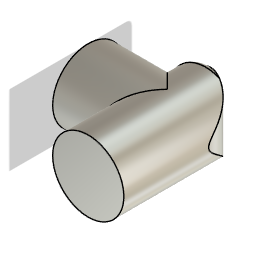
Link5 v14 (Autodesk Fusion 360 design; units mm, degrees)
Autodesk Fusion 360 part; units mm, degrees
sketch "Boceto1" plane through (0, 0, 0) normal (0, 0, 1) x (1, 0, 0)
  circle A0 centre (0, 0) radius 45
  circle A1 centre (0, 0) radius 30
  dimension "d1" = 90
  dimension "d12" = 60
  constraint coincident A0.centre A1.centre
  measures "d1" diameter of A0
  measures "d12" diameter of A1
extrude "Extruir1" add sketch "Boceto1" along normal blind 100 contours A0 | A1
sketch "Boceto2" plane through (0, 0, 0) normal (1, 0, 0) x (0, 0, -1)
  circle A0 centre (0, 0) radius 45
  circle A1 centre (0, 0) radius 32.5
  dimension "d4" = 90
  dimension "d15" = 65
  constraint coincident A0.centre A1.centre
  measures "d4" diameter of A0
  measures "d15" diameter of A1
  measures "d21" distance of A0.centre
extrude "Extruir2" add sketch "Boceto2" along normal blind 55.5 and the other way blind 100 contours A0 | A1
fillet "Empalme1" radius 7 1 edges at (55.5, -16.2727, 41.9547)
sketch "Sketch3" plane through (0, 0, 0) normal (0, 1, 0) x (1, 0, 0)
  spline S0 degree 5 poles (57.3838, -29.8061) (56.8787, -19.3252) (55.0357, -0.6641) (49.7748, 20.4314) (38.231, 36.7866) (17.1828, 45.0023) (-5.2478, 46.7966) (-25.9392, 47.254) (-41.6586, 47.3556) (-50, 47.3556) knots 0 0 0 0 0 0 0.2 0.4 0.6 0.8 1 1 1 1 1 1
  line L0 (-30, 47.3556) -> (-70, 47.3556)
  line L1 (58.498, -52.9268) -> (56.2695, -6.6855)
  line L2 (57.3838, -29.8061) -> (57.3838, 47.3556)
  line L3 (57.3838, 47.3556) -> (-50, 47.3556)
  constraint midpoint S0.end L0
  constraint midpoint S0.start L1
  constraint perpendicular L0 L2
  constraint perpendicular L2 L3
extrude "Extrude3" cut sketch "Sketch3" along normal through all and the other way through all
extrude "Extrude4" cut sketch "Boceto1" along normal blind 80 contours A1
extrude "Extrude5" cut sketch "Boceto2" against normal blind 85 contours A1
move_body "Desplazar1" bodies 1 to x (0, 0, -1) y (-1, 0, 0) z (0, 1, 0) at (15, 0, 15)
move_body "Desplazar2" bodies 1 to x (1, 0, 0) y (0, 0, -1) z (0, 1, 0) at (0, 85, 115)
move_body "Desplazar3" bodies 1 to x (1, 0, 0) y (0, 1, 0) z (0, 0, 1) at (0, -50, -90)
move_body "Desplazar4" bodies 1 to x (1, 0, 0) y (0, 0, -1) z (0, 1, 0) at (0, 125, -25)
move_body "Desplazar5" bodies 1 to x (0, 0, -1) y (0, 1, 0) z (1, 0, 0) at (75, 0, -45)
move_body "Desplazar6" bodies 1 to x (0, -1, 0) y (1, 0, 0) z (0, 0, 1) at (-50, 50, 0)
move_body "Desplazar7" bodies 1 to x (1, 0, 0) y (0, 1, 0) z (0, 0, 1) at (0, -5, 15)
move_body "Move8" bodies 1 to x (0, 1, 0) y (-1, 0, 0) z (0, 0, 1) at (96.5, -103.5, 0)
move_body "Move9" bodies 1 to x (-1, 0, 0) y (0, 1, 0) z (0, 0, -1) at (200, 0, -90)
move_body "Move10" bodies 1 to x (1, 0, 0) y (0, 1, 0) z (0, 0, 1) at (-150, 103.5, 45)
sketch "Sketch4" plane through (0, 0, 0) normal (0, 1, 0) x (1, 0, 0)
  line L0 (0, 0) -> (0, 90)
  constraint coincident L0.start origin
  constraint vertical L0
sketch "Sketch5" plane through (98.5, 0, 0) normal (1, 0, 0) x (0, 0, -1)
  circle A0 centre (0, 100) radius 45
  line L0 (0, -103.5) -> (0, 0)
  dimension "d21" = 103.5
  constraint coincident L0.end origin
  constraint vertical L0
  measures "d21" distance of L0.end L0.start
sketch "Sketch6" plane through (0, 0, 0) normal (0, 0, 1) x (1, 0, 0)
  point P0 (98.5, 100)
  dimension "d22" = 100
  dimension "d23" = 98.5
  measures "d22" vertical distance of P0 origin
  measures "d23" horizontal distance of P0 origin
